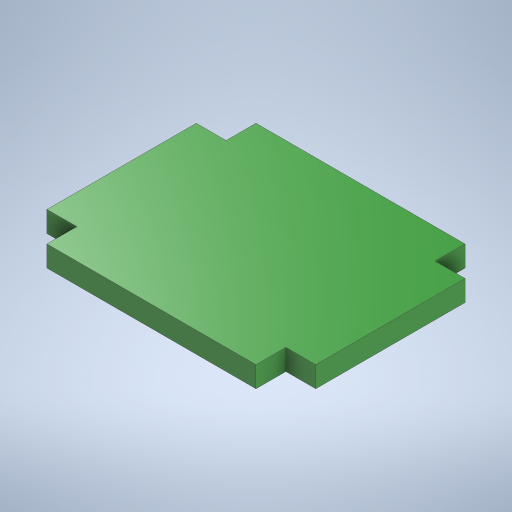
# Autodesk Inventor part: pcb
Saved by Autodesk Inventor 2024.1 (Build 281209000, 209)
## iProperties
Created: 2023-10-24
Part Number: pcb
Material: Générique
Document SubType Name: Modeling
Designer: Thibault
Density: 1 g/cm^3
Appearance: Par défaut
Author: Thibault
Autodesk Inventor part; units mm, degrees
ref_plane "YZ Plane" through (0, 0, 0) normal (1, 0, 0) x (0, 1, 0)
ref_plane "XZ Plane" through (0, 0, 0) normal (0, 1, 0) x (-1, 0, 0)
ref_plane "XY Plane" through (0, 0, 0) normal (0, 0, 1) x (1, 0, 0)
sketch "Esquisse1" plane through (0, 0, 0) normal (0, 1, 0) x (-1, 0, 0)
  line L0 (4.9536, 5.2597) -> (4.9536, 3.2597)
  line L1 (4.9536, 3.2597) -> (6.9536, 3.2597)
  line L2 (-9.0464, 5.2597) -> (-9.0464, 3.2597)
  line L3 (-9.0464, 3.2597) -> (-11.0464, 3.2597)
  line L4 (-9.0464, -8.7403) -> (-9.0464, -6.7403)
  line L5 (-9.0464, -6.7403) -> (-11.0464, -6.7403)
  line L6 (4.9536, -8.7403) -> (4.9536, -6.7403)
  line L7 (4.9536, -6.7403) -> (6.9536, -6.7403)
  line L8 (4.9536, 5.2597) -> (-9.0464, 5.2597)
  line L9 (-11.0464, 3.2597) -> (-11.0464, -6.7403)
  line L10 (-9.0464, -8.7403) -> (4.9536, -8.7403)
  line L11 (6.9536, -6.7403) -> (6.9536, 3.2597)
  point P0 (0, 0)
  dimension "d2" = 2
  dimension "d3" = 2
  dimension "d4" = 2
  dimension "d5" = 2
  dimension "d6" = 2
  dimension "d7" = 2
  dimension "d8" = 2
  dimension "d9" = 2
  dimension "d16" = 10
  dimension "d17" = 18
  constraints: 24 end point, 9 perpendicular, 2 parallel, 1 horizontal
  measures "d2" distance of L1.end L0.end
  measures "d3" distance of L0.end L0.start
  measures "d4" distance of L2.end L3.end
  measures "d5" distance of L2.start L2.end
  measures "d6" distance of L5.end L4.end
  measures "d7" distance of L4.end L4.start
  measures "d8" distance of L6.end L7.end
  measures "d9" distance of L6.start L6.end
  measures "d16" distance of L4.end L2.end
  measures "d17" distance between parallel lines of L11 L9
extrude "Extrusion1" add sketch "Esquisse1" along normal blind 1.4
